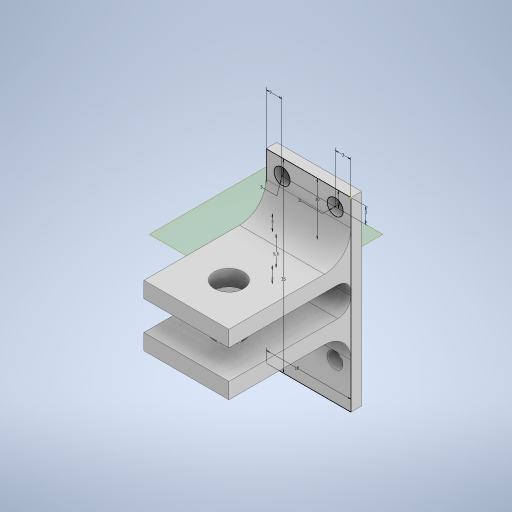
# Autodesk Inventor part: держатель вала
Saved by Autodesk Inventor 2024.2 (Build 282272000, 272)
## iProperties
Created: 2025-11-27
Part Number: держатель вала
Material: Типовые
Document SubType Name: Modeling
Designer: Zakhar
Density: 1 g/cm^3
Appearance: По умолчанию
Author: Zakhar
Autodesk Inventor part; units mm, degrees
ref_plane "YZ Plane" through (0, 0, 0) normal (1, 0, 0) x (0, 1, 0)
ref_plane "XZ Plane" through (0, 0, 0) normal (0, 1, 0) x (-1, 0, 0)
ref_plane "XY Plane" through (0, 0, 0) normal (0, 0, 1) x (1, 0, 0)
sketch "Эскиз6" plane through (0, 0, 0) normal (0, 0, 1) x (1, 0, 0)
  line L0 (0, 0) -> (-16, 0)
  line L1 (-16, 0) -> (-16, -35)
  line L2 (-16, -35) -> (0, -35)
  line L3 (0, -35) -> (0, 0)
  circle A0 centre (-3, -3) radius 1.5
  circle A1 centre (-13, -3) radius 1.5
  line L4 (0, -10) -> (-16, -10)
  line L5 (-16, -10) -> (-16, -35)
  line L6 (-16, -35) -> (0, -35)
  line L7 (0, -35) -> (0, -10)
  line L8 (0, -13) -> (-16, -13)
  line L9 (0, -18.5) -> (-16, -18.5)
  line L10 (-16, -21.5) -> (0, -21.5)
  point P0 (-16, -10)
  point P1 (0, -21.5)
  dimension "d42" = 16
  dimension "d43" = 35
  dimension "d44" = 3
  dimension "d45" = 3
  dimension "d46" = 3
  dimension "d47" = 3
  dimension "d48" = 3
  dimension "d49" = 3
  dimension "d59" = 10
  dimension "d60" = 3
  dimension "d61" = 3
  dimension "d62" = 5.5
  constraints: 22 end point, 7 point on line, 5 perpendicular, 4 parallel, 2 centre point, 2 horizontal, 1 coincident
  measures "d42" distance of L1.end L2.end
  measures "d43" distance of L0.end L1.end
  measures "d44" diameter of A1
  measures "d45" diameter of A0
  measures "d46" distance from line of L0 A1.centre
  measures "d47" distance from line of L1 A1.centre
  measures "d48" distance from line of L0 A0.centre
  measures "d49" distance from line of L3 A0.centre
  measures "d59" distance between parallel lines of L0 L4
  measures "d60" distance between parallel lines of L4 L8
  measures "d61" distance between parallel lines of L10 L9
  measures "d62" distance between parallel lines of L9 L8
extrude "Выдавливание8" add sketch "Эскиз6" against normal blind 2 contours L3 L4 L1 L0
ref_plane "РабПлоскость12" through (-16, -14, 0) normal (0, -1, 0) x (1, 0, 0)
sketch "Эскиз7" plane through (-16, -14, 0) normal (0, -1, 0) x (1, 0, 0)
  line L0 (0, 0) -> (16, 0) projected
  line L1 (16, -2) -> (0, -2) projected
  circle A0 centre (8, 15) radius 2.75
  point P0 (8, 0)
  dimension "d56" = 5.5
  dimension "d71" = 15
  constraints: 1 centre point, 1 midpoint
  measures "d56" diameter of A0
  measures "d71" distance from line of A0.centre L0
extrude "Выдавливание11" add sketch "Эскиз6" along normal blind 23 contours L3 L8 L1 L4 | L3 L10 L1 L9
extrude "Выдавливание12" add sketch "Эскиз6" against normal blind 2 contours L3 L8 L1 L4 | L3 L9 L1 L8 | L3 L10 L1 L9 | L3 L2 L1 L10
fillet "Сопряжение грани1" radius 5 1 edges at (-8, -10, 0)
fillet "Сопряжение грани2" radius 2.5 1 edges at (-8, -13, 0)
fillet "Сопряжение грани3" radius 5 2 edges at (-8, -18.5, 0) (-8, -21.5, 0)
fillet "Сопряжение1" radius 2.5 1 edges at (-8, -18.5, 0)
extrude "Выдавливание13" cut sketch "Эскиз7" along normal mid plane 24
sketch "Эскиз8" plane through (0, 0, -2) normal (0, 0, -1) x (-1, 0, 0)
  line L0 (16, -35) -> (16, 0) projected
  line L1 (16, 0) -> (0, 0) projected
  line L2 (0, 0) -> (0, -35) projected
  line L3 (0, -35) -> (16, -35) projected
  circle A0 centre (3, -3) radius 1.5 projected
  circle A1 centre (13, -3) radius 1.5 projected
  circle A2 centre (13, -28) radius 1.5
  circle A3 centre (3, -28) radius 1.5
  dimension "d74" = 3
  dimension "d76" = 3
  dimension "d77" = 25
  dimension "d78" = 3
  dimension "d79" = 25
  constraints: 2 centre point, 1 equal radius
  measures "d74" diameter of A2
  measures "d76" distance from line of A2.centre L0
  measures "d77" distance of A1.centre A2.centre
  measures "d78" distance from line of L2 A3.centre
  measures "d79" distance of A0.centre A3.centre
extrude "Выдавливание14" cut sketch "Эскиз8" against normal through all contours A2 | A3
